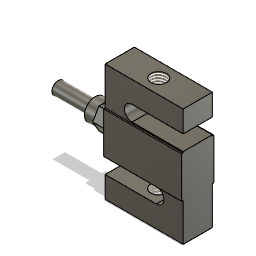
Load Cell (300 kg) v1 (Autodesk Fusion 360 design; units mm, degrees)
Autodesk Fusion 360 part; units mm, degrees
sketch "Sketch1" plane through (0, 0, 0) normal (0, 0, 1) x (1, 0, 0)
  line L0 (0, 0) -> (50.75, 0)
  line L1 (50.75, 0) -> (50.75, 52.25)
  line L2 (50.75, 52.25) -> (12.5, 52.25)
  line L3 (12.5, 52.25) -> (12.5, 62.25)
  line L4 (12.5, 62.25) -> (50.75, 62.25)
  line L5 (50.75, 62.25) -> (50.75, 76.25)
  line L6 (50.75, 76.25) -> (0, 76.25)
  line L7 (0, 76.25) -> (0, 24)
  line L8 (0, 24) -> (38.25, 24)
  line L9 (38.25, 24) -> (38.25, 14)
  line L10 (38.25, 14) -> (0, 14)
  line L11 (0, 14) -> (0, 0)
  line L12 (0, 24.75) -> (50.75, 24.75)
  line L13 (50.75, 51.5) -> (0, 51.5)
  dimension "d1" = 76.25
  dimension "d2" = 14
  dimension "d3" = 10
  dimension "d4" = 50.75
  dimension "d5" = 12.5
  dimension "d6" = 0.75
  dimension "d7" = 0.75
  constraint coincident L0.start L11.end
  constraint horizontal L0
  constraint perpendicular L0 L1
  constraint perpendicular L1 L2
  constraint perpendicular L2 L3
  constraint perpendicular L3 L4
  constraint perpendicular L4 L5
  constraint perpendicular L5 L6
  constraint perpendicular L6 L7
  constraint perpendicular L7 L8
  constraint perpendicular L8 L9
  constraint perpendicular L9 L10
  constraint perpendicular L0 L11
  constraint equal L5 L11
  constraint equal L3 L9
  constraint collinear L7 L11
  constraint collinear L1 L5
  constraint equal L2 L10
  constraint coincident L7 L12.start
  constraint coincident L1 L12.end
  constraint perpendicular L1 L12
  constraint coincident L1 L13.start
  constraint coincident L7 L13.end
  constraint perpendicular L7 L13
  measures "d1" distance of L0 L6
  measures "d2" distance of L4.end L5.end
  measures "d3" distance of L2.end L3.end
  measures "d4" distance of L5.end L6.end
  measures "d5" distance of L1 L9
  measures "d6" distance of L8 L12
  measures "d7" distance of L2 L13
extrude "Extrude1" add sketch "Sketch1" along normal mid plane 19
extrude "Extrude2" add sketch "Sketch1" along normal mid plane 21 contours L1 L7 L12 L13
sketch "Sketch2" plane through (0, 0, 0) normal (-1, 0, 0) x (0, 0, 1)
  line L0 (9.5, 51.5) -> (9.5, 76.25)
  line L1 (9.5, 76.25) -> (-9.5, 76.25)
  line L2 (-9.5, 76.25) -> (-9.5, 51.5)
  line L3 (-9.5, 51.5) -> (-10.5, 51.5)
  line L4 (-10.5, 51.5) -> (-10.5, 24.75)
  line L5 (-10.5, 24.75) -> (-9.5, 24.75)
  line L6 (-9.5, 24.75) -> (-9.5, 24)
  line L7 (-9.5, 24) -> (9.5, 24)
  line L8 (9.5, 24) -> (9.5, 24.75)
  line L9 (9.5, 24.75) -> (10.5, 24.75)
  line L10 (10.5, 24.75) -> (10.5, 51.5)
  line L11 (10.5, 51.5) -> (9.5, 51.5)
  line L12 (8.0829, 38.125) -> (4.0415, 45.125)
  line L13 (4.0415, 45.125) -> (-4.0415, 45.125)
  line L14 (-4.0415, 45.125) -> (-8.0829, 38.125)
  line L15 (-8.0829, 38.125) -> (-4.0415, 31.125)
  line L16 (-4.0415, 31.125) -> (4.0415, 31.125)
  line L17 (4.0415, 31.125) -> (8.0829, 38.125)
  line L18 (-9.5, 0) -> (9.5, 0)
  line L19 (0, 76.25) -> (0, 24)
  circle A0 centre (0, 38.125) radius 4.1
  circle A1 centre (0, 38.125) radius 7
  point P0 (0, 38.125)
  dimension "d12" = 7
  dimension "d13" = 38.125
  dimension "d14" = 8.2
  dimension "d15" = 14
  constraint horizontal L16
  constraint coincident P0 L19
  constraint coincident P0 A0.centre
  constraint concentric A0 A1
  measures "d12" distance of P0 L17
  measures "d13" distance of P0 L18
  measures "d14" diameter of A0
  measures "d15" diameter of A1
extrude "Extrude3" add sketch "Sketch2" along normal blind 9.5 contours L13 L14 A1 | L19 A0 A1 | L12 L13 A1 | L19 A0 A1 | L19 A0 | L19 A0 | L12 L17 A1 | L14 L15 A1 | L15 L16 A1 | L16 L17 A1
extrude "Extrude4" add sketch "Sketch2" along normal blind 16 contours L19 A0 A1 | L19 A0 A1 | L19 A0 | L19 A0
extrude "Extrude5" add sketch "Sketch2" along normal blind 40 contours L19 A0 | L19 A0
fillet "Fillet1" radius 5 4 edges at (38.25, 14, 0) (38.25, 24, 0) (12.5, 62.25, 0) (12.5, 52.25, 0)
sketch "Sketch3" plane through (0, 76.25, 0) normal (0, 1, 0) x (-1, 0, 0)
  line L0 (0, -9.5) -> (0, 9.5)
  line L1 (0, 9.5) -> (-50.75, 9.5)
  line L2 (-50.75, 9.5) -> (-50.75, -9.5)
  line L3 (-50.75, -9.5) -> (0, -9.5)
  circle A0 centre (-25.375, 0) radius 6
  line L4 (0, 4.0415) -> (0, -4.0415)
  line L5 (-50.75, 0) -> (0, 0)
  dimension "d24" = 25.375
  dimension "d25" = 12
  constraint coincident A0.centre L5
  measures "d24" distance of A0.centre L4
  measures "d25" diameter of A0
extrude "Extrude6" cut sketch "Sketch3" against normal up to surface (14 mm away) contours A0 L5 | A0 L5
extrude "Extrude7" cut sketch "Sketch3" along normal up to surface (14 mm away) from surface at -76.25 contours A0 L5 | A0 L5
thread "Thread1" "ISO Metric profile 12.0 M12x1.75 6H" major diameter 12.2265 minor diameter 10.2735 pitch 1.75 angle 60 resizes the face on face at (19.3825, 66.9167, -0.2991)
thread "Thread2" "ISO Metric profile 12.0 M12x1.75 6H" major diameter 12.2265 minor diameter 10.2735 pitch 1.75 angle 60 resizes the face on face at (19.4048, 4.6667, -0.5974)
equation "d8 = ( 19 / 2 ) * 1 mm"
equation "d10 = ( 21 / 2 ) * 1 mm"
equation "d12 = ( 14 / 2 ) * 1 mm"
equation "d13 = d1 / 2"
equation "d24 = d4 / 2"
